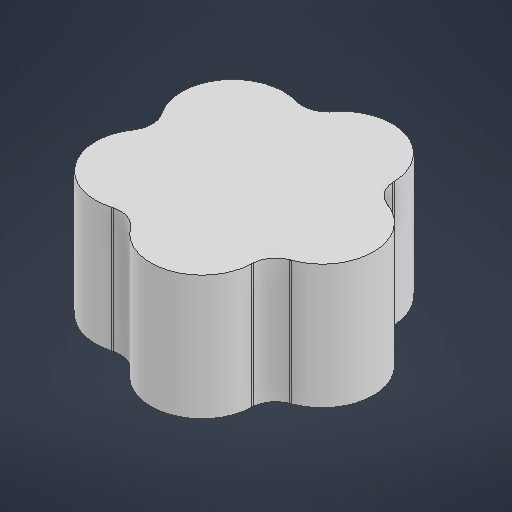
# Autodesk Inventor part: Flower
Saved by Autodesk Inventor 2026.2 (Build 302298000, 298)
## iProperties
Created: 2026-02-17
Part Number: Flower
Material: Generic
Document SubType Name: Modeling
Designer: mayhe
Density: 1 g/cm^3
Appearance: Default
Author: mayhe
Autodesk Inventor part; units mm, degrees
ref_plane "YZ Plane" through (0, 0, 0) normal (1, 0, 0) x (0, 1, 0)
ref_plane "XZ Plane" through (0, 0, 0) normal (0, 1, 0) x (-1, 0, 0)
ref_plane "XY Plane" through (0, 0, 0) normal (0, 0, 1) x (1, 0, 0)
sketch "Sketch1" plane through (0, 0, 0) normal (0, 1, 0) x (-1, 0, 0)
  line L0 (-1.7898, 0.9776) -> (-1.8283, 0.965)
  line L1 (-1.4828, 1.4406) -> (-1.4828, 1.4001)
  arc A0 (0.3766, 2.0042) -> (-1.4828, 1.4001) centre (-0.4549, 1.4001) ccw
  line L2 (0.3766, 2.0042) -> (0.3528, 2.037)
  line L3 (0.9119, 1.8554) -> (0.8734, 1.8429)
  arc A1 (2.0225, 0.2611) -> (0.8734, 1.8429) centre (1.191, 0.8653) ccw
  line L4 (2.0225, 0.2611) -> (2.0463, 0.2939)
  line L5 (2.0463, -0.2939) -> (2.0225, -0.2611)
  arc A2 (0.8734, -1.8429) -> (2.0225, -0.2611) centre (1.191, -0.8653) ccw
  line L6 (0.8734, -1.8429) -> (0.9119, -1.8554)
  line L7 (0.3528, -2.037) -> (0.3766, -2.0042)
  arc A3 (-1.4828, -1.4001) -> (0.3766, -2.0042) centre (-0.4549, -1.4001) ccw
  line L8 (-1.4828, -1.4001) -> (-1.4828, -1.4406)
  line L9 (-1.8283, -0.965) -> (-1.7898, -0.9776)
  arc A4 (-1.7898, 0.9776) -> (-1.7898, -0.9776) centre (-1.4721, 0) ccw
  arc A5 (0.3528, 2.037) -> (0.9119, 1.8554) centre (0.7574, 2.3309) ccw
  arc A6 (-1.8283, 0.965) -> (-1.4828, 1.4406) centre (-1.9828, 1.4406) ccw
  arc A7 (-1.4828, -1.4406) -> (-1.8283, -0.965) centre (-1.9828, -1.4406) ccw
  arc A8 (0.9119, -1.8554) -> (0.3528, -2.037) centre (0.7574, -2.3309) ccw
  arc A9 (2.0463, 0.2939) -> (2.0463, -0.2939) centre (2.4508, 0) ccw
  point P0 (0, 0)
  point P1 (0, 0)
  point P2 (2.5, 0)
  point P3 (2.5, -1.8164)
  point P4 (-0.9549, -2.9389)
  point P5 (-3.0902, 0)
  point P6 (-0.9549, 2.9389)
  point P7 (2.5, 1.8164)
  dimension "d6" = 0.5
  constraints: 20 end point, 20 point on circle, 10 centre point, 10 tangent, 4 equal radius, 6 other
  measures "d6" radius of A5
extrude "Extrusion1" add sketch "Sketch1" along normal mid plane 2.5
body "Solid1"
